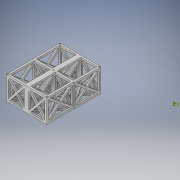
# Autodesk Inventor part: 4 Tape Measures Holder 2
Saved by Autodesk Inventor 2019 (Build 230136000, 136)
## iProperties
Created: 2019-01-03
Part Number: 4 Tape Measures Holder 2
Material: Generic
Document SubType Name: Modeling
Designer: ashle
Density: 1 g/cm^3
Appearance: Default
TM1W: 51.500 mm
TM1L: 70.000 mm
TM1H: 77.000 mm
TM2W: 50.500 mm
TM2L: 71.000 mm
TM2H: 74.200 mm
uw: 6.000 mm
HS: 15.000 mm
VS: 6.500 mm
TM1THL: 130.000 mm
TM2THL: 128.000 mm
TM1TVL: 85.250 mm
TM2TVL: 86.250 mm
Screw: 3.900 mm
Author: ashle
Autodesk Inventor part; units mm, degrees
ref_plane "YZ Plane" through (0, 0, 0) normal (1, 0, 0) x (0, 1, 0)
sketch "Sketch1" plane through (0, 0, 0) normal (0, 1, 0) x (-1, 0, 0)
  line L0 (59, -79.25) -> (7.5, -79.25) construction
  line L1 (7.5, -79.25) -> (7.5, -3.25) construction
  line L2 (7.5, -3.25) -> (59, -3.25) construction
  line L3 (59, -3.25) -> (59, -79.25) construction
  line L4 (-7.5, -79.25) -> (-59, -79.25) construction
  line L5 (-59, -79.25) -> (-59, -3.25) construction
  line L6 (-59, -3.25) -> (-7.5, -3.25) construction
  line L7 (-7.5, -3.25) -> (-7.5, -79.25) construction
  line L8 (58, 3.25) -> (7.5, 3.25) construction
  line L9 (7.5, 3.25) -> (7.5, 80.25) construction
  line L10 (7.5, 80.25) -> (58, 80.25) construction
  line L11 (58, 80.25) -> (58, 3.25) construction
  line L12 (-7.5, 3.25) -> (-58, 3.25) construction
  line L13 (-58, 3.25) -> (-58, 80.25) construction
  line L14 (-58, 80.25) -> (-7.5, 80.25) construction
  line L15 (-7.5, 80.25) -> (-7.5, 3.25) construction
  line L16 (65, -85.25) -> (-65, -85.25)
  line L17 (-65, -85.25) -> (-65, 0)
  line L18 (65, 0) -> (65, -85.25)
  line L19 (-64, 0) -> (-64, 86.25)
  line L20 (-64, 86.25) -> (64, 86.25)
  line L21 (64, 86.25) -> (64, 0)
  line L22 (210.5449, 0) -> (-191.5447, 0) construction
  line L23 (0, -253.0755) -> (0, 334.1089) construction
  line L24 (-65, 0) -> (-64, 0)
  line L25 (64, 0) -> (65, 0)
  line L26 (59, -3.25) -> (7.5, -79.25) construction
  line L27 (59, -79.25) -> (7.5, -3.25) construction
  line L28 (-7.5, -79.25) -> (-59, -3.25) construction
  line L29 (-59, -79.25) -> (-7.5, -3.25) construction
  line L30 (7.5, 3.25) -> (58, 80.25) construction
  line L31 (58, 3.25) -> (7.5, 80.25) construction
  line L32 (-7.5, 80.25) -> (-58, 3.25) construction
  line L33 (-7.5, 3.25) -> (-58, 80.25) construction
  line L34 (61.4835, -4.9329) -> (56.5165, -1.5671) construction
  line L35 (56.5165, -1.5671) -> (5.0165, -77.5671) construction
  line L36 (5.0165, -77.5671) -> (9.9835, -80.9329) construction
  line L37 (9.9835, -80.9329) -> (61.4835, -4.9329) construction
  line L38 (56.5165, -80.9329) -> (61.4835, -77.5671) construction
  line L39 (61.4835, -77.5671) -> (9.9835, -1.5671) construction
  line L40 (9.9835, -1.5671) -> (5.0165, -4.9329) construction
  line L41 (5.0165, -4.9329) -> (56.5165, -80.9329) construction
  line L42 (33.25, -46.5979) -> (11.1239, -79.25)
  line L43 (7.5, -73.9021) -> (29.6261, -41.25)
  line L44 (33.25, -46.5979) -> (55.3761, -79.25)
  line L45 (59, -73.9021) -> (36.8739, -41.25)
  line L46 (36.8739, -41.25) -> (59, -8.5979)
  line L47 (55.3761, -3.25) -> (33.25, -35.9021)
  line L48 (33.25, -35.9021) -> (11.1239, -3.25)
  line L49 (7.5, -8.5979) -> (29.6261, -41.25)
  line L50 (55.3761, -79.25) -> (11.1239, -79.25)
  line L51 (7.5, -73.9021) -> (7.5, -8.5979)
  line L52 (11.1239, -3.25) -> (55.3761, -3.25)
  line L53 (59, -8.5979) -> (59, -73.9021)
  line L54 (-9.9835, -80.9329) -> (-61.4835, -4.9329) construction
  line L55 (-61.4835, -4.9329) -> (-56.5165, -1.5671) construction
  line L56 (-56.5165, -1.5671) -> (-5.0165, -77.5671) construction
  line L57 (-5.0165, -77.5671) -> (-9.9835, -80.9329) construction
  line L58 (-56.5165, -80.9329) -> (-61.4835, -77.5671) construction
  line L59 (-61.4835, -77.5671) -> (-9.9835, -1.5671) construction
  line L60 (-9.9835, -1.5671) -> (-5.0165, -4.9329) construction
  line L61 (-5.0165, -4.9329) -> (-56.5165, -80.9329) construction
  line L62 (-55.3761, -79.25) -> (-33.25, -46.5979)
  line L63 (-33.25, -46.5979) -> (-11.1239, -79.25)
  line L64 (-7.5, -73.9021) -> (-29.6261, -41.25)
  line L65 (-29.6261, -41.25) -> (-7.5, -8.5979)
  line L66 (-7.5, -8.5979) -> (-7.5, -73.9021)
  line L67 (-11.1239, -79.25) -> (-55.3761, -79.25)
  line L68 (-59, -73.9021) -> (-36.8739, -41.25)
  line L69 (-36.8739, -41.25) -> (-59, -8.5979)
  line L70 (-59, -8.5979) -> (-59, -73.9021)
  line L71 (-33.25, -35.9021) -> (-55.3761, -3.25)
  line L72 (-55.3761, -3.25) -> (-11.1239, -3.25)
  line L73 (-11.1239, -3.25) -> (-33.25, -35.9021)
  line L74 (-4.9914, 4.8953) -> (-10.0086, 1.6047) construction
  line L75 (-10.0086, 1.6047) -> (-60.5086, 78.6047) construction
  line L76 (-60.5086, 78.6047) -> (-55.4914, 81.8953) construction
  line L77 (-55.4914, 81.8953) -> (-4.9914, 4.8953) construction
  line L78 (-55.4914, 1.6047) -> (-60.5086, 4.8953) construction
  line L79 (-60.5086, 4.8953) -> (-10.0086, 81.8953) construction
  line L80 (-10.0086, 81.8953) -> (-4.9914, 78.6047) construction
  line L81 (-4.9914, 78.6047) -> (-55.4914, 1.6047) construction
  line L82 (-11.0876, 3.25) -> (-54.4124, 3.25)
  line L83 (-54.4124, 3.25) -> (-32.75, 36.2797)
  line L84 (-32.75, 36.2797) -> (-11.0876, 3.25)
  line L85 (-7.5, 8.7203) -> (-29.1624, 41.75)
  line L86 (-29.1624, 41.75) -> (-7.5, 74.7797)
  line L87 (-7.5, 74.7797) -> (-7.5, 8.7203)
  line L88 (-32.75, 47.2203) -> (-11.0876, 80.25)
  line L89 (-11.0876, 80.25) -> (-54.4124, 80.25)
  line L90 (-54.4124, 80.25) -> (-32.75, 47.2203)
  line L91 (-36.3376, 41.75) -> (-58, 8.7203)
  line L92 (-58, 8.7203) -> (-58, 74.7797)
  line L93 (-58, 74.7797) -> (-36.3376, 41.75)
  line L94 (55.4914, 1.6047) -> (60.5086, 4.8953) construction
  line L95 (60.5086, 4.8953) -> (10.0086, 81.8953) construction
  line L96 (10.0086, 81.8953) -> (4.9914, 78.6047) construction
  line L97 (4.9914, 78.6047) -> (55.4914, 1.6047) construction
  line L98 (10.0086, 1.6047) -> (4.9914, 4.8953) construction
  line L99 (4.9914, 4.8953) -> (55.4914, 81.8953) construction
  line L100 (55.4914, 81.8953) -> (60.5086, 78.6047) construction
  line L101 (60.5086, 78.6047) -> (10.0086, 1.6047) construction
  line L102 (58, 74.7797) -> (36.3376, 41.75)
  line L103 (36.3376, 41.75) -> (58, 8.7203)
  line L104 (58, 8.7203) -> (58, 74.7797)
  line L105 (54.4124, 80.25) -> (32.75, 47.2203)
  line L106 (32.75, 47.2203) -> (11.0876, 80.25)
  line L107 (11.0876, 80.25) -> (54.4124, 80.25)
  line L108 (7.5, 74.7797) -> (29.1624, 41.75)
  line L109 (7.5, 8.7203) -> (29.1624, 41.75)
  line L110 (7.5, 8.7203) -> (7.5, 74.7797)
  line L111 (54.4124, 3.25) -> (11.0876, 3.25)
  line L112 (11.0876, 3.25) -> (32.75, 36.2797)
  line L113 (32.75, 36.2797) -> (54.4124, 3.25)
  point P0 (0, 86.25)
  point P1 (0, -85.25)
  point P2 (0, 0)
  dimension "TM1HL" = 130
  dimension "TM2HL" = 128
  dimension "TM1STV" = 85.25
  dimension "TM2STV" = 86.25
  dimension "d26" = 6
  dimension "d27" = 6
  dimension "d31" = 6
  dimension "d32" = 6
  dimension "d33" = 6
  dimension "d34" = 6
  dimension "d37" = 6.5
  dimension "d38" = 6.5
  dimension "d39" = 15
  dimension "d40" = 15
  dimension "d41" = 7.5
  dimension "d42" = 7.5
  dimension "d45" = 3.25
  dimension "d46" = 3.25
  dimension "d47" = 6
  dimension "d49" = 6
  dimension "d50" = 6
  dimension "d51" = 6
  dimension "d52" = 6
  dimension "d53" = 6
  dimension "d54" = 6
  dimension "d55" = 6
  dimension "d56" = 6
  dimension "d57" = 6
  constraints: 228 end point, 100 point on line, 37 parallel, 18 midpoint, 17 collinear, 16 perpendicular, 7 horizontal, 2 vertical, 1 other
  measures "TM1HL" distance of L16.start L16.end
  measures "TM2HL" distance of L19.end L20.end
  measures "TM1STV" distance of L18.start L16.start
  measures "TM2STV" distance of L21.end L20.end
  measures "d26" distance between parallel lines of L18 L3
  measures "d27" distance between parallel lines of L17 L5
  measures "d31" distance between parallel lines of L21 L11
  measures "d32" distance between parallel lines of L20 L10
  measures "d33" distance between parallel lines of L20 L14
  measures "d34" distance between parallel lines of L19 L13
  measures "d37" distance between parallel lines of L8 L2
  measures "d38" distance between parallel lines of L6 L12
  measures "d39" distance between parallel lines of L7 L1
  measures "d40" distance between parallel lines of L15 L9
  measures "d41" distance between parallel lines of L23 L15
  measures "d42" distance between parallel lines of L23 L7
  measures "d45" distance between parallel lines of L2 L22
  measures "d46" distance between parallel lines of L6 L22
  measures "d47" distance between parallel lines of L35 L37
  measures "d49" distance between parallel lines of L41 L39
  measures "d50" distance between parallel lines of L16 L0
  measures "d51" distance between parallel lines of L16 L4
  measures "d52" distance between parallel lines of L54 L56
  measures "d53" distance between parallel lines of L59 L61
  measures "d54" distance between parallel lines of L75 L77
  measures "d55" distance between parallel lines of L79 L81
  measures "d56" distance between parallel lines of L97 L95
  measures "d57" distance between parallel lines of L99 L101
extrude "Base Extrusion" add sketch "Sketch1" along normal blind 6
sketch "Sketch4" plane through (-64, 0, 86.25) normal (0, 0, 1) x (1, 0, 0)
  line L0 (0, 0) -> (128, 0)
  line L1 (128, 0) -> (128, 74.2)
  line L2 (128, 74.2) -> (0, 74.2)
  line L3 (0, 74.2) -> (0, 0)
  line L4 (128, 0) -> (0, 0) projected
  line L5 (0, 0) -> (0, 6) projected
  line L6 (128, 0) -> (128, 6) projected
  line L7 (6, 68.2) -> (56.5, 68.2) construction
  line L8 (56.5, 68.2) -> (56.5, 6) construction
  line L9 (56.5, 6) -> (6, 6) construction
  line L10 (6, 6) -> (6, 68.2) construction
  line L11 (71.5, 68.2) -> (122, 68.2) construction
  line L12 (122, 68.2) -> (122, 6) construction
  line L13 (122, 6) -> (71.5, 6) construction
  line L14 (71.5, 6) -> (71.5, 68.2) construction
  line L15 (0, 6) -> (128, 6) projected
  line L16 (6, 68.2) -> (56.5, 6) construction
  line L17 (3.671, 66.3091) -> (8.329, 70.0909) construction
  line L18 (8.329, 70.0909) -> (58.829, 7.8909) construction
  line L19 (58.829, 7.8909) -> (54.171, 4.1091) construction
  line L20 (54.171, 4.1091) -> (3.671, 66.3091) construction
  line L21 (56.5, 68.2) -> (6, 6) construction
  line L22 (54.171, 70.0909) -> (58.829, 66.3091) construction
  line L23 (58.829, 66.3091) -> (8.329, 4.1091) construction
  line L24 (8.329, 4.1091) -> (3.671, 7.8909) construction
  line L25 (3.671, 7.8909) -> (54.171, 70.0909) construction
  line L26 (6, 10.7596) -> (27.3857, 37.1)
  line L27 (27.3857, 37.1) -> (6, 63.4404)
  line L28 (6, 63.4404) -> (6, 10.7596)
  line L29 (129, 6) -> (-1, 6) projected
  line L30 (9.8643, 6) -> (31.25, 32.3404)
  line L31 (31.25, 32.3404) -> (52.6357, 6)
  line L32 (52.6357, 6) -> (9.8643, 6)
  line L33 (52.8761, 0) -> (52.8761, 6) projected
  line L34 (56.5, 10.7596) -> (35.1143, 37.1)
  line L35 (35.1143, 37.1) -> (56.5, 63.4404)
  line L36 (56.5, 63.4404) -> (56.5, 10.7596)
  line L37 (31.25, 41.8596) -> (52.6357, 68.2)
  line L38 (9.8643, 68.2) -> (52.6357, 68.2)
  line L39 (9.8643, 68.2) -> (31.25, 41.8596)
  line L40 (71.5, 68.2) -> (122, 6) construction
  line L41 (69.171, 66.3091) -> (73.829, 70.0909) construction
  line L42 (73.829, 70.0909) -> (124.329, 7.8909) construction
  line L43 (124.329, 7.8909) -> (119.671, 4.1091) construction
  line L44 (119.671, 4.1091) -> (69.171, 66.3091) construction
  line L45 (71.5, 6) -> (122, 68.2) construction
  line L46 (69.171, 7.8909) -> (73.829, 4.1091) construction
  line L47 (73.829, 4.1091) -> (124.329, 66.3091) construction
  line L48 (124.329, 66.3091) -> (119.671, 70.0909) construction
  line L49 (119.671, 70.0909) -> (69.171, 7.8909) construction
  line L50 (71.5, 63.4404) -> (92.8857, 37.1)
  line L51 (92.8857, 37.1) -> (71.5, 10.7596)
  line L52 (71.5, 10.7596) -> (71.5, 63.4404)
  line L53 (75.1239, 0) -> (75.1239, 6) projected
  line L54 (75.1239, 6) -> (96.75, 32.3404)
  line L55 (96.75, 32.3404) -> (118.1357, 6)
  line L56 (119.3761, 6) -> (97.25, 6) projected
  line L57 (118.1357, 6) -> (75.1239, 6)
  line L58 (100.6143, 37.1) -> (122, 63.4404)
  line L59 (122, 63.4404) -> (122, 10.7596)
  line L60 (100.6143, 37.1) -> (122, 10.7596)
  line L61 (75.3643, 68.2) -> (96.75, 41.8596)
  line L62 (96.75, 41.8596) -> (118.1357, 68.2)
  line L63 (118.1357, 68.2) -> (75.3643, 68.2)
  point P0 (64, 0)
  dimension "d77" = 74.2
  dimension "d78" = 6
  dimension "d79" = 6
  dimension "d80" = 6
  dimension "d81" = 6
  dimension "d82" = 15
  dimension "d83" = 50.5
  dimension "d84" = 50.5
  dimension "d85" = 6
  dimension "d86" = 6
  dimension "d87" = 6
  dimension "d88" = 6
  constraints: 112 end point, 45 point on line, 19 parallel, 9 collinear, 9 perpendicular, 8 midpoint, 3 horizontal, 1 vertical, 3 other
  measures "d77" distance of L0.end L1.end
  measures "d78" distance between parallel lines of L2 L7
  measures "d79" distance between parallel lines of L3 L10
  measures "d80" distance between parallel lines of L2 L11
  measures "d81" distance between parallel lines of L1 L12
  measures "d82" distance between parallel lines of L14 L8
  measures "d83" distance of L7.start L7.end
  measures "d84" distance of L11.start L11.end
  measures "d85" distance between parallel lines of L20 L18
  measures "d86" distance between parallel lines of L23 L25
  measures "d87" distance between parallel lines of L42 L44
  measures "d88" distance between parallel lines of L49 L47
extrude "TM2L Outer" add sketch "Sketch4" against normal up to surface (6 mm away) contours L3 L2 L1 L15 L55 L54 L31 L30
sketch "Sketch5" plane through (65, 0, -85.25) normal (0, 0, -1) x (-1, 0, 0)
  line L0 (0, 0) -> (130, 0)
  line L1 (130, 0) -> (130, 74.2)
  line L2 (130, 74.2) -> (0, 74.2)
  line L3 (0, 74.2) -> (0, 0)
  line L4 (130, 0) -> (0, 0) projected
  line L5 (130, 0) -> (130, 6) projected
  line L6 (0, 0) -> (0, 6) projected
  line L7 (6, 68.2) -> (57.5, 68.2) construction
  line L8 (57.5, 68.2) -> (57.5, 6) construction
  line L9 (57.5, 6) -> (6, 6) construction
  line L10 (6, 6) -> (6, 68.2) construction
  line L11 (72.5, 68.2) -> (124, 68.2) construction
  line L12 (124, 68.2) -> (124, 6) construction
  line L13 (124, 6) -> (72.5, 6) construction
  line L14 (72.5, 6) -> (72.5, 68.2) construction
  line L15 (0, 6) -> (130, 6) projected
  line L16 (6, 68.2) -> (57.5, 6) construction
  line L17 (3.6893, 66.2868) -> (8.3107, 70.1132) construction
  line L18 (8.3107, 70.1132) -> (59.8107, 7.9132) construction
  line L19 (59.8107, 7.9132) -> (55.1893, 4.0868) construction
  line L20 (55.1893, 4.0868) -> (3.6893, 66.2868) construction
  line L21 (57.5, 68.2) -> (6, 6) construction
  line L22 (55.1893, 70.1132) -> (59.8107, 66.2868) construction
  line L23 (59.8107, 66.2868) -> (8.3107, 4.0868) construction
  line L24 (8.3107, 4.0868) -> (3.6893, 7.9132) construction
  line L25 (3.6893, 7.9132) -> (55.1893, 70.1132) construction
  line L26 (9.8949, 68.2) -> (53.6051, 68.2)
  line L27 (53.6357, 68.2) -> (10.8643, 68.2) projected
  line L28 (53.6051, 68.2) -> (31.75, 41.8041)
  line L29 (31.75, 41.8041) -> (9.8949, 68.2)
  line L30 (6, 63.4959) -> (27.8551, 37.1)
  line L31 (27.8551, 37.1) -> (6, 10.7041)
  line L32 (6, 10.7041) -> (6, 63.4959)
  line L33 (9.8949, 6) -> (31.75, 32.3959)
  line L34 (31.75, 32.3959) -> (53.6051, 6)
  line L35 (53.9124, 6) -> (10.5876, 6) projected
  line L36 (53.6051, 6) -> (9.8949, 6)
  line L37 (35.6449, 37.1) -> (57.5, 63.4959)
  line L38 (57.5, 63.4959) -> (57.5, 10.7041)
  line L39 (57.5, 10.7041) -> (35.6449, 37.1)
  line L40 (124, 68.2) -> (72.5, 6) construction
  line L41 (72.5, 68.2) -> (124, 6) construction
  line L42 (70.1893, 66.2868) -> (74.8107, 70.1132) construction
  line L43 (74.8107, 70.1132) -> (126.3107, 7.9132) construction
  line L44 (126.3107, 7.9132) -> (121.6893, 4.0868) construction
  line L45 (121.6893, 4.0868) -> (70.1893, 66.2868) construction
  line L46 (121.6893, 70.1132) -> (126.3107, 66.2868) construction
  line L47 (126.3107, 66.2868) -> (74.8107, 4.0868) construction
  line L48 (74.8107, 4.0868) -> (70.1893, 7.9132) construction
  line L49 (70.1893, 7.9132) -> (121.6893, 70.1132) construction
  line L50 (98.25, 41.8041) -> (120.1051, 68.2)
  line L51 (120.1051, 68.2) -> (76.3949, 68.2)
  line L52 (76.3949, 68.2) -> (98.25, 41.8041)
  line L53 (102.1449, 37.1) -> (124, 63.4959)
  line L54 (124, 63.4959) -> (124, 10.7041)
  line L55 (124, 10.7041) -> (102.1449, 37.1)
  line L56 (98.25, 32.3959) -> (120.1051, 6)
  line L57 (120.1051, 6) -> (76.3949, 6)
  line L58 (76.1239, 6) -> (120.3761, 6) projected
  line L59 (76.3949, 6) -> (98.25, 32.3959)
  line L60 (94.3551, 37.1) -> (72.5, 10.7041)
  line L61 (72.5, 10.7041) -> (72.5, 63.4959)
  line L62 (72.5, 63.4959) -> (94.3551, 37.1)
  point P0 (65, 0)
  point P1 (101.8757, 6)
  point P2 (20.2911, 6)
  dimension "d92" = 74.2
  dimension "d93" = 6
  dimension "d94" = 6
  dimension "d95" = 15
  dimension "d96" = 51.5
  dimension "d97" = 51.5
  dimension "d98" = 6
  dimension "d99" = 6
  dimension "d100" = 6
  dimension "d101" = 6
  dimension "d102" = 6
  dimension "d103" = 6
  constraints: 112 end point, 48 point on line, 18 parallel, 12 collinear, 8 midpoint, 7 perpendicular, 3 horizontal
  measures "d92" distance of L2.end L0.start
  measures "d93" distance between parallel lines of L3 L10
  measures "d94" distance between parallel lines of L2 L7
  measures "d95" distance between parallel lines of L14 L8
  measures "d96" distance of L7.start L7.end
  measures "d97" distance of L11.start L11.end
  measures "d98" distance between parallel lines of L1 L12
  measures "d99" distance between parallel lines of L2 L11
  measures "d100" distance between parallel lines of L18 L20
  measures "d101" distance between parallel lines of L23 L25
  measures "d102" distance between parallel lines of L43 L45
  measures "d103" distance between parallel lines of L47 L49
extrude "TM1L Outer" add sketch "Sketch5" against normal up to surface (6 mm away) contours L3 L2 L1 L15 L56 L59 L34 L33
sketch "Sketch7" plane through (-54.4124, 0, 3.25) normal (0, 0, 1) x (1, 0, 0)
  line L0 (-9.5876, 74.2) -> (118.4124, 74.2)
  line L1 (118.4124, 74.2) -> (118.4124, 0)
  line L2 (118.4124, 0) -> (-9.5876, 0)
  line L3 (-9.5876, 0) -> (-9.5876, 74.2)
  line L4 (118.4124, 0) -> (-9.5876, 0) projected
  line L5 (118.4124, 0) -> (118.4124, 74.2) projected
  line L6 (-9.5876, 0) -> (-9.5876, 74.2) projected
  line L7 (118.4124, 74.2) -> (-9.5876, 74.2) projected
  line L8 (0.2766, 68.2) -> (21.6624, 41.8596)
  line L9 (0.2766, 68.2) -> (43.0481, 68.2)
  line L10 (43.0481, 68.2) -> (21.6624, 41.8596)
  line L11 (-3.5876, 63.4404) -> (-3.5876, 10.7596)
  line L12 (-3.5876, 10.7596) -> (17.7981, 37.1)
  line L13 (17.7981, 37.1) -> (-3.5876, 63.4404)
  line L14 (21.6624, 32.3404) -> (0.2766, 6)
  line L15 (0.2766, 6) -> (43.0481, 6)
  line L16 (21.6624, 32.3404) -> (43.0481, 6)
  line L17 (17.7981, 37.1) -> (-3.5876, 10.7596) projected
  line L18 (-3.5876, 63.4404) -> (17.7981, 37.1) projected
  line L19 (-3.5876, 10.7596) -> (-3.5876, 63.4404) projected
  line L20 (21.6624, 41.8596) -> (0.2766, 68.2) projected
  line L21 (0.2766, 68.2) -> (43.0481, 68.2) projected
  line L22 (43.0481, 68.2) -> (21.6624, 41.8596) projected
  line L23 (21.6624, 32.3404) -> (43.0481, 6) projected
  line L24 (0.2766, 6) -> (43.0481, 6) projected
  line L25 (0.2766, 6) -> (21.6624, 32.3404) projected
  line L26 (25.5266, 37.1) -> (46.9124, 63.4404)
  line L27 (46.9124, 63.4404) -> (46.9124, 10.7596)
  line L28 (46.9124, 10.7596) -> (25.5266, 37.1)
  line L29 (25.5266, 37.1) -> (46.9124, 63.4404) projected
  line L30 (46.9124, 10.7596) -> (25.5266, 37.1) projected
  line L31 (46.9124, 63.4404) -> (46.9124, 10.7596) projected
  line L32 (61.9124, 63.4404) -> (83.2981, 37.1)
  line L33 (83.2981, 37.1) -> (61.9124, 10.7596)
  line L34 (61.9124, 10.7596) -> (61.9124, 63.4404)
  line L35 (65.7766, 68.2) -> (87.1624, 41.8596)
  line L36 (87.1624, 41.8596) -> (108.5481, 68.2)
  line L37 (108.5481, 68.2) -> (65.7766, 68.2)
  line L38 (114.9615, 66.5802) -> (91.0266, 37.1)
  line L39 (91.0266, 37.1) -> (112.4124, 10.7596)
  line L40 (112.4124, 10.7596) -> (112.4124, 63.4404)
  line L41 (87.1624, 32.3404) -> (65.5363, 6)
  line L42 (65.5363, 6) -> (108.5481, 6)
  line L43 (108.5481, 6) -> (87.1624, 32.3404)
  line L44 (61.9124, 63.4404) -> (83.2981, 37.1) projected
  line L45 (83.2981, 37.1) -> (61.9124, 10.7596) projected
  line L46 (61.9124, 10.7596) -> (61.9124, 63.4404) projected
  line L47 (87.1624, 41.8596) -> (65.7766, 68.2) projected
  line L48 (65.7766, 68.2) -> (108.5481, 68.2) projected
  line L49 (108.5481, 68.2) -> (87.1624, 41.8596) projected
  line L50 (91.0266, 37.1) -> (112.4124, 63.4404) projected
  line L51 (112.4124, 63.4404) -> (112.4124, 10.7596) projected
  line L52 (112.4124, 10.7596) -> (91.0266, 37.1) projected
  line L53 (87.1624, 32.3404) -> (108.5481, 6) projected
  line L54 (65.5363, 6) -> (87.1624, 32.3404) projected
  line L55 (65.5363, 6) -> (108.5481, 6) projected
  point P0 (54.4124, 0)
  constraints: 56 end point, 28 collinear, 2 horizontal, 2 parallel, 2 perpendicular, 1 point on line, 1 vertical
extrude "Horizontal Barrier TM2" add sketch "Sketch7" against normal up to surface (3.25 mm away)
sketch "Sketch10" plane through (64, 74.2, 0) normal (0, 0, -1) x (-1, 0, 0)
  line L0 (-1, 0) -> (129, 0)
  line L1 (129, 0) -> (129, -68.2)
  line L2 (129, -68.2) -> (-1, -68.2)
  line L3 (-1, -68.2) -> (-1, 0)
  line L4 (75.3643, -68.2) -> (52.8761, -68.2)
  line L5 (129, -74.2) -> (129, 0) projected
  line L6 (-1, -74.2) -> (-1, 0) projected
  line L7 (128, 0) -> (0, 0) projected
  line L8 (-9.5945, -82.6479) -> (27.3857, -37.1)
  line L9 (9.8643, -6) -> (31.25, -32.3404)
  line L10 (31.25, -32.3404) -> (52.6357, -6)
  line L11 (52.6357, -6) -> (9.8643, -6)
  line L12 (56.5, -10.7596) -> (35.1143, -37.1)
  line L13 (35.1143, -37.1) -> (56.5, -63.4404)
  line L14 (56.5, -63.4404) -> (56.5, -10.7596)
  line L15 (31.25, -41.8596) -> (9.8643, -68.2)
  line L16 (9.8643, -68.2) -> (52.8761, -68.2)
  line L17 (52.8761, -68.2) -> (31.25, -41.8596)
  line L18 (71.5, -10.7596) -> (71.5, -63.4404)
  line L19 (71.5, -63.4404) -> (92.8857, -37.1)
  line L20 (92.8857, -37.1) -> (71.5, -10.7596)
  line L21 (75.3643, -6) -> (96.75, -32.3404)
  line L22 (96.75, -32.3404) -> (118.1357, -6)
  line L23 (118.1357, -6) -> (75.3643, -6)
  line L24 (122, -10.7596) -> (100.6143, -37.1)
  line L25 (100.6143, -37.1) -> (122, -63.4404)
  line L26 (122, -63.4404) -> (122, -10.7596)
  line L27 (96.75, -41.8596) -> (75.3643, -68.2)
  line L28 (75.3643, -68.2) -> (118.1357, -68.2)
  line L29 (118.1357, -68.2) -> (96.75, -41.8596)
  line L30 (6, -10.7596) -> (6, -57.2402)
  line L31 (6, -57.2402) -> (6, -63.4404)
  line L32 (6, -63.4404) -> (27.3857, -37.1)
  line L33 (27.3857, -37.1) -> (6, -10.7596)
  line L34 (6, -10.7596) -> (27.3857, -37.1) projected
  line L35 (6, -63.4404) -> (6, -10.7596) projected
  line L36 (27.3857, -37.1) -> (6, -63.4404) projected
  line L37 (31.25, -32.3404) -> (9.8643, -6) projected
  line L38 (9.8643, -6) -> (52.6357, -6) projected
  line L39 (52.6357, -6) -> (31.25, -32.3404) projected
  line L40 (35.1143, -37.1) -> (56.5, -10.7596) projected
  line L41 (56.5, -10.7596) -> (56.5, -63.4404) projected
  line L42 (56.5, -63.4404) -> (35.1143, -37.1) projected
  line L43 (31.25, -41.8596) -> (52.8761, -68.2) projected
  line L44 (9.8643, -68.2) -> (31.25, -41.8596) projected
  line L45 (52.8761, -68.2) -> (9.8643, -68.2) projected
  line L46 (75.3643, -68.2) -> (96.75, -41.8596) projected
  line L47 (96.75, -41.8596) -> (118.1357, -68.2) projected
  line L48 (100.6143, -37.1) -> (122, -10.7596) projected
  line L49 (122, -63.4404) -> (100.6143, -37.1) projected
  line L50 (122, -10.7596) -> (122, -63.4404) projected
  line L51 (75.3643, -6) -> (118.1357, -6) projected
  line L52 (118.1357, -6) -> (96.75, -32.3404) projected
  line L53 (96.75, -32.3404) -> (75.3643, -6) projected
  line L54 (71.5, -10.7596) -> (92.8857, -37.1) projected
  line L55 (71.5, -63.4404) -> (71.5, -10.7596) projected
  line L56 (92.8857, -37.1) -> (71.5, -63.4404) projected
  point P0 (64, -74.2)
  constraints: 62 end point, 28 collinear, 4 point on line, 1 horizontal, 1 parallel, 1 perpendicular
extrude "Horizontal Barrier TM1" add sketch "Sketch10" along normal up to surface (3.25 mm away) contours L0 L1 L2 L29 L27 L17 L15 L3
sketch "Sketch11" plane through (-65, 0, -85.25) normal (-1, 0, 0) x (0, 0, 1)
  line L0 (0, 74.2) -> (85.25, 74.2)
  line L1 (85.25, 74.2) -> (85.25, 0)
  line L2 (85.25, 0) -> (0, 0)
  line L3 (0, 0) -> (0, 74.2)
  line L4 (0, 0) -> (0, 74.2) projected
  line L5 (85.25, 0) -> (0, 0) projected
  line L6 (85.25, 0) -> (85.25, 74.2) projected
  line L7 (85.25, 74.2) -> (82, 74.2) projected
  line L8 (6, 68.2) -> (82, 68.2) construction
  line L9 (82, 68.2) -> (82, 6) construction
  line L10 (82, 6) -> (6, 6) construction
  line L11 (6, 6) -> (6, 68.2) construction
  line L12 (6, 74.2) -> (6, 6) projected
  line L13 (6, 6) -> (82, 6) projected
  line L14 (82, 6) -> (82, 74.2) projected
  line L15 (49.3479, 6) -> (82, 6) construction
  line L16 (6, 68.2) -> (82, 6) construction
  line L17 (6, 6) -> (6, 32.3959) construction
  line L18 (82, 68.2) -> (6, 6) construction
  line L19 (4.1, 65.8784) -> (7.9, 70.5216) construction
  line L20 (7.9, 70.5216) -> (83.9, 8.3216) construction
  line L21 (83.9, 8.3216) -> (80.1, 3.6784) construction
  line L22 (80.1, 3.6784) -> (4.1, 65.8784) construction
  line L23 (80.1, 70.5216) -> (83.9, 65.8784) construction
  line L24 (83.9, 65.8784) -> (7.9, 3.6784) construction
  line L25 (7.9, 3.6784) -> (4.1, 8.3216) construction
  line L26 (4.1, 8.3216) -> (80.1, 70.5216) construction
  line L27 (10.7367, 68.2) -> (44, 40.9766)
  line L28 (44, 40.9766) -> (77.2633, 68.2)
  line L29 (77.2633, 68.2) -> (10.7367, 68.2)
  line L30 (6, 64.3234) -> (6, 9.8766)
  line L31 (6, 9.8766) -> (39.2633, 37.1)
  line L32 (39.2633, 37.1) -> (6, 64.3234)
  line L33 (82, 64.3234) -> (48.7367, 37.1)
  line L34 (48.7367, 37.1) -> (82, 9.8766)
  line L35 (82, 9.8766) -> (82, 64.3234)
  line L36 (44, 33.2234) -> (10.7367, 6)
  line L37 (10.7367, 6) -> (77.2633, 6)
  line L38 (77.2633, 6) -> (44, 33.2234)
  dimension "d118" = 6
  dimension "d119" = 6
  dimension "d120" = 6
  constraints: 60 end point, 19 collinear, 10 parallel, 4 midpoint, 4 perpendicular, 2 horizontal
  measures "d118" distance between parallel lines of L0 L8
  measures "d119" distance between parallel lines of L20 L22
  measures "d120" distance between parallel lines of L24 L26
extrude "TM1 Left Side" add sketch "Sketch11" against normal up to surface (6 mm away) contours L0 L12 L13 L14 L1 L2 L3 | L0 L14 L33 L34 L13 L38 L36 L12 L31 L32
ref_plane "Center of TM1HS" through (0, 0, -8.5979) normal (1, 0, 0) x (0, 0, -1)
mirror "TM1 Right Side" about plane through (0, 0, -8.5979) normal (1, 0, 0) of "TM1 Left Side"
sketch "Sketch12" plane through (64, 0, 86.25) normal (1, 0, 0) x (0, 0, -1)
  line L0 (0, 74.2) -> (86.25, 74.2)
  line L1 (86.25, 74.2) -> (86.25, 0)
  line L2 (86.25, 0) -> (0, 0)
  line L3 (0, 0) -> (0, 74.2)
  line L4 (86.25, 0) -> (0, 0) projected
  line L5 (0, 0) -> (0, 74.2) projected
  line L6 (86.25, 0) -> (86.25, 74.2) projected
  line L7 (83, 74.2) -> (86.25, 74.2) projected
  line L8 (6, 68.2) -> (83, 68.2) construction
  line L9 (83, 68.2) -> (83, 6) construction
  line L10 (83, 6) -> (6, 6) construction
  line L11 (6, 6) -> (6, 68.2) construction
  line L12 (6, 74.2) -> (6, 6) construction
  line L13 (6, 6) -> (83, 6) construction
  line L14 (83, 6) -> (83, 74.2) construction
  line L15 (6, 68.2) -> (83, 6) construction
  line L16 (6, 0) -> (6, 6) construction
  line L17 (6, 6) -> (83, 68.2) construction
  line L18 (4.1148, 65.8663) -> (7.8852, 70.5337) construction
  line L19 (7.8852, 70.5337) -> (84.8852, 8.3337) construction
  line L20 (84.8852, 8.3337) -> (81.1148, 3.6663) construction
  line L21 (81.1148, 3.6663) -> (4.1148, 65.8663) construction
  line L22 (81.1148, 70.5337) -> (84.8852, 65.8663) construction
  line L23 (84.8852, 65.8663) -> (7.8852, 3.6663) construction
  line L24 (7.8852, 3.6663) -> (4.1148, 8.3337) construction
  line L25 (4.1148, 8.3337) -> (81.1148, 70.5337) construction
  line L26 (10.7741, 68.2) -> (44.5, 40.9565)
  line L27 (44.5, 40.9565) -> (78.2259, 68.2)
  line L28 (78.2259, 68.2) -> (10.7741, 68.2)
  line L29 (6, 64.3435) -> (6, 9.8565)
  line L30 (6, 9.8565) -> (39.7259, 37.1)
  line L31 (39.7259, 37.1) -> (6, 64.3435)
  line L32 (44.5, 33.2435) -> (10.7741, 6)
  line L33 (10.7741, 6) -> (78.2259, 6)
  line L34 (78.2259, 6) -> (44.5, 33.2435)
  line L35 (83, 64.3435) -> (49.2741, 37.1)
  line L36 (49.2741, 37.1) -> (83, 9.8565)
  line L37 (83, 9.8565) -> (83, 64.3435)
  dimension "d124" = 6
  dimension "d125" = 6
  dimension "d126" = 6
  constraints: 61 end point, 19 collinear, 10 parallel, 4 midpoint, 4 perpendicular, 2 horizontal, 1 vertical
  measures "d124" distance between parallel lines of L0 L8
  measures "d125" distance between parallel lines of L21 L19
  measures "d126" distance between parallel lines of L23 L25
extrude "TM2 Right Side" add sketch "Sketch12" against normal up to surface (6 mm away)
ref_plane "Center of TM2HS" through (0, 0, 8.7203) normal (-1, 0, 0) x (0, 0, 1)
mirror "TM2 Left Side" about plane through (0, 0, 8.7203) normal (-1, 0, 0) of "TM2 Right Side"
sketch "Sketch13" plane through (-7.5, 0, 74.7797) normal (-1, 0, 0) x (0, 0, 1)
  line L0 (-74.7797, 74.2) -> (11.4703, 74.2)
  line L1 (11.4703, 74.2) -> (11.4703, 0)
  line L2 (11.4703, 0) -> (-74.7797, 0)
  line L3 (-74.7797, 0) -> (-74.7797, 74.2)
  line L4 (11.4703, 74.2) -> (-74.7797, 74.2) projected
  line L5 (11.4703, 0) -> (11.4703, 74.2) projected
  line L6 (-74.7797, 0) -> (-74.7797, 74.2) projected
  line L7 (11.4703, 0) -> (-74.7797, 0) projected
  line L8 (-71.5297, 68.2) -> (5.4703, 68.2) construction
  line L9 (5.4703, 68.2) -> (5.4703, 6) construction
  line L10 (5.4703, 6) -> (-71.5297, 6) construction
  line L11 (-71.5297, 6) -> (-71.5297, 68.2) construction
  line L12 (0.6961, 68.2) -> (-66.7556, 68.2) construction
  line L13 (5.4703, 9.8565) -> (5.4703, 64.3435) construction
  line L14 (-66.7556, 6) -> (0.6961, 6) construction
  line L15 (-71.5297, 64.3435) -> (-71.5297, 9.8565) construction
  line L16 (-71.5297, 68.2) -> (-71.5297, 41.8596) construction
  line L17 (-71.5297, 68.2) -> (5.4703, 6) construction
  line L18 (5.4703, 68.2) -> (-71.5297, 6) construction
  line L19 (-73.4149, 65.8663) -> (-69.6446, 70.5337) construction
  line L20 (-69.6446, 70.5337) -> (7.3554, 8.3337) construction
  line L21 (7.3554, 8.3337) -> (3.5851, 3.6663) construction
  line L22 (3.5851, 3.6663) -> (-73.4149, 65.8663) construction
  line L23 (3.5851, 70.5337) -> (7.3554, 65.8663) construction
  line L24 (7.3554, 65.8663) -> (-69.6446, 3.6663) construction
  line L25 (-69.6446, 3.6663) -> (-73.4149, 8.3337) construction
  line L26 (-73.4149, 8.3337) -> (3.5851, 70.5337) construction
  line L27 (-66.7556, 68.2) -> (-33.0297, 40.9565)
  line L28 (-33.0297, 40.9565) -> (0.6961, 68.2)
  line L29 (0.6961, 68.2) -> (-66.7556, 68.2)
  line L30 (5.4703, 64.3435) -> (-28.2556, 37.1)
  line L31 (-28.2556, 37.1) -> (5.4703, 9.8565)
  line L32 (5.4703, 9.8565) -> (5.4703, 64.3435)
  line L33 (-33.0297, 33.2435) -> (-66.7556, 6)
  line L34 (-66.7556, 6) -> (0.6961, 6)
  line L35 (0.6961, 6) -> (-33.0297, 33.2435)
  line L36 (-66.0595, 6) -> (0, 6) projected
  line L37 (-71.5297, 64.3435) -> (-71.5297, 9.8565)
  line L38 (-71.5297, 9.8565) -> (-37.8039, 37.1)
  line L39 (-37.8039, 37.1) -> (-71.5297, 64.3435)
  line L40 (-71.5297, 63.4404) -> (-71.5297, 10.7596) projected
  dimension "d130" = 6
  dimension "d131" = 6
  constraints: 60 end point, 20 collinear, 10 parallel, 4 horizontal, 4 midpoint, 4 perpendicular, 1 vertical
  measures "d130" distance between parallel lines of L24 L26
  measures "d131" distance between parallel lines of L20 L22
extrude "TM2 Vertical Barrier" add sketch "Sketch13" against normal up to surface (15 mm away)
sketch "Sketch14" plane through (-7.5, 0, -8.5979) normal (-1, 0, 0) x (0, 0, 1)
  line L0 (-76.6521, 74.2) -> (8.5979, 74.2)
  line L1 (8.5979, 74.2) -> (8.5979, 0)
  line L2 (8.5979, 0) -> (-76.6521, 0)
  line L3 (-76.6521, 0) -> (-76.6521, 74.2)
  line L4 (-76.6521, 74.2) -> (8.5979, 74.2) projected
  line L5 (8.5979, 0) -> (8.5979, 74.2) projected
  line L6 (8.5979, 0) -> (-76.6521, 0) projected
  line L7 (-76.6521, 0) -> (-76.6521, 74.2) projected
  line L8 (-65.9154, 68.2) -> (-32.6521, 40.9766)
  line L9 (-32.6521, 40.9766) -> (0.6112, 68.2)
  line L10 (0.6112, 68.2) -> (-65.9154, 68.2)
  line L11 (-70.6521, 64.3234) -> (-70.6521, 9.8766)
  line L12 (-70.6521, 9.8766) -> (-37.3888, 37.1)
  line L13 (-37.3888, 37.1) -> (-70.6521, 64.3234)
  line L14 (-32.6521, 33.2234) -> (-65.9154, 6)
  line L15 (-65.9154, 6) -> (0.6112, 6)
  line L16 (0.6112, 6) -> (-32.6521, 33.2234)
  line L17 (5.3479, 64.3234) -> (-27.9154, 37.1)
  line L18 (5.3479, 9.8766) -> (5.3479, 64.3234)
  line L19 (-27.9154, 37.1) -> (5.3479, 9.8766)
  line L20 (-70.6521, 64.3234) -> (-37.3888, 37.1) projected
  line L21 (-37.3888, 37.1) -> (-70.6521, 9.8766) projected
  line L22 (-70.6521, 64.3234) -> (-70.6521, 9.8766) projected
  line L23 (-65.9154, 68.2) -> (0.6112, 68.2) projected
  line L24 (0.6112, 68.2) -> (-32.6521, 40.9766) projected
  line L25 (-32.6521, 40.9766) -> (-65.9154, 68.2) projected
  line L26 (-27.9154, 37.1) -> (5.3479, 64.3234) projected
  line L27 (5.3479, 9.8766) -> (5.3479, 64.3234) projected
  line L28 (5.3479, 9.8766) -> (-27.9154, 37.1) projected
  line L29 (-32.6521, 33.2234) -> (0.6112, 6) projected
  line L30 (-65.9154, 6) -> (-32.6521, 33.2234) projected
  line L31 (-65.9154, 6) -> (0.6112, 6) projected
  constraints: 32 end point, 16 collinear, 3 point on line, 2 parallel, 2 perpendicular, 1 horizontal, 1 vertical
extrude "TM1 Vertical Barrier" add sketch "Sketch14" against normal up to surface (15 mm away)
sketch "Sketch15" plane through (-64, 74.2, 86.25) normal (0, 1, 0) x (1, 0, 0)
  circle A0 centre (2, 168.5) radius 1.95
  line L0 (-1, 171.5) -> (129, 171.5) construction
  line L1 (-1, 171.5) -> (5, 171.5) construction
  line L2 (5, 171.5) -> (5, 165.5) construction
  line L3 (5, 165.5) -> (-1, 165.5) construction
  line L4 (-1, 165.5) -> (-1, 171.5) construction
  line L5 (2, 168.5) -> (2, 171.5) construction
  line L6 (2, 168.5) -> (2, 165.5) construction
  line L7 (2, 168.5) -> (-1, 168.5) construction
  line L8 (2, 168.5) -> (5, 168.5) construction
  line L9 (64, 194.995) -> (64, -20.5528) construction
  circle A1 centre (126, 168.5) radius 1.95
  line L10 (129, 171.5) -> (123, 171.5) construction
  line L11 (123, 171.5) -> (123, 165.5) construction
  line L12 (123, 165.5) -> (129, 165.5) construction
  line L13 (129, 165.5) -> (129, 171.5) construction
  line L14 (126, 168.5) -> (126, 171.5) construction
  line L15 (126, 168.5) -> (126, 165.5) construction
  line L16 (126, 168.5) -> (129, 168.5) construction
  line L17 (126, 168.5) -> (123, 168.5) construction
  circle A2 centre (64, 86.25) radius 1.95
  line L18 (0, 6) -> (6, 6) construction
  line L19 (6, 6) -> (6, 0) construction
  line L20 (6, 0) -> (0, 0) construction
  line L21 (0, 0) -> (0, 6) construction
  line L22 (0, 0) -> (0, 86.25) construction
  line L23 (128, 0) -> (0, 0) construction
  line L24 (6, 6) -> (6, 83) construction
  line L25 (6, 6) -> (56.5, 6) construction
  circle A3 centre (3, 3) radius 1.95
  line L26 (3, 3) -> (3, 6) construction
  line L27 (3, 3) -> (6, 3) construction
  line L28 (3, 3) -> (3, 0) construction
  line L29 (3, 3) -> (0, 3) construction
  line L30 (128, 6) -> (122, 6) construction
  line L31 (122, 6) -> (122, 0) construction
  line L32 (122, 0) -> (128, 0) construction
  line L33 (128, 0) -> (128, 6) construction
  circle A4 centre (125, 3) radius 1.95
  line L34 (125, 3) -> (125, 6) construction
  line L35 (125, 3) -> (122, 3) construction
  line L36 (125, 3) -> (125, 0) construction
  line L37 (125, 3) -> (128, 3) construction
  point P0 (122, 6)
  dimension "d136" = 3.9
  dimension "d137" = 3.9
  dimension "d138" = 3.9
  constraints: 66 end point, 19 symmetric about line, 9 point on line, 8 collinear, 8 midpoint, 5 centre point, 4 parallel, 3 perpendicular, 2 horizontal, 2 vertical, 1 coincident, 2 other
  measures "d136" diameter of A0
  measures "d137" diameter of A2
  measures "d138" diameter of A3
extrude "Top Screw Holes" cut sketch "Sketch15" against normal blind 6
sketch "Sketch17" plane through (0, 0, 0) normal (0, -1, 0) x (1, 0, 0)
  circle A0 centre (-62, -82.25) radius 1.95 projected
  circle A1 centre (-62, -82.25) radius 1.95
  circle A2 centre (62, -82.25) radius 1.95 projected
  circle A3 centre (62, -82.25) radius 1.95
  circle A4 centre (61, 83.25) radius 1.95 projected
  circle A5 centre (61, 83.25) radius 1.95
  circle A6 centre (-61, 83.25) radius 1.95 projected
  circle A7 centre (-61, 83.25) radius 1.95
  constraints: 4 centre point, 4 coincident
extrude "Extrusion16" cut sketch "Sketch17" against normal blind 6
equation "\"d26\" = uw"
equation "\"d27\" = uw"
equation "\"d31\" = uw"
equation "\"d32\" = uw"
equation "\"d33\" = uw"
equation "\"d34\" = uw"
equation "\"d37\" = VS"
equation "\"d38\" = VS"
equation "\"d39\" = HS"
equation "\"d40\" = HS"
equation "\"d41\" = 0.5 * HS"
equation "\"d42\" = 0.5 * HS"
equation "\"d45\" = 0.5 * VS"
equation "\"d46\" = 0.5 * VS"
equation "\"d47\" = uw"
equation "\"d49\" = uw"
equation "\"TM1W\" = 51.5"
equation "\"TM1L\" = 70"
equation "\"TM1H\" = 77"
equation "\"TM2W\" = 50.5"
equation "\"TM2L\" = 71"
equation "\"TM2H\" = 74.2"
equation "\"uw\" = 6"
equation "\"HS\" = 15"
equation "\"VS\" = 6.5"
equation "\"TM1THL\" = 130"
equation "\"TM2THL\" = 128"
equation "\"TM1TVL\" = 85.25"
equation "\"TM2TVL\" = 86.25"
equation "\"Screw\" = 3.9"
body "Solid1"
